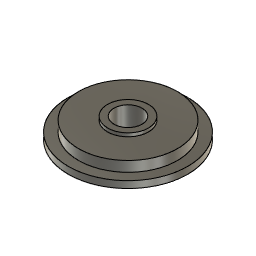
Spaced Boss v2 (Autodesk Fusion 360 design; units mm, degrees)
Autodesk Fusion 360 part; units mm, degrees
sketch "Sketch1" plane through (0, 0, 0) normal (0, 0, 1) x (1, 0, 0)
  circle A0 centre (0, 0) radius 14.5
  circle A1 centre (0, 0) radius 17.5
  dimension "d1" = 29
  dimension "d10" = 35
  constraint coincident A0.centre A1.centre
  constraint concentric A0 A1
  measures "d1" diameter of A0
  measures "d10" diameter of A1
extrude "Extrude1" add sketch "Sketch1" along normal blind 3 contours A0
sketch "Sketch2" plane through (0, 0, 3) normal (0, 0, 1) x (-1, 0, 0)
  circle A0 centre (0, 0) radius 14.5
  circle A1 centre (0, 0) radius 4.1
  circle A2 centre (0, 0) radius 6
  dimension "d4" = 8.2
  dimension "d5" = 12
  constraint coincident A0.centre A1.centre
  constraint concentric A1 A2
  measures "d4" diameter of A1
  measures "d5" diameter of A2
extrude "Extrude2" add sketch "Sketch2" along normal blind 1 contours A2
extrude "Extrude3" cut 1 faces at (1.5011, -0.3426, 3) along direction (0, 0, -1) blind 10
extrude "Extrude4" add sketch "Sketch1" against normal blind 2 contours A0 | A1
extrude "Extrude5" cut 1 faces at (1.5011, -0.3426, 0) along direction (0, 0, -1) blind 17.993
